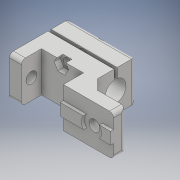
# Autodesk Inventor part: EixoXY - Canto
Saved by Autodesk Inventor 2017 (Build 210142000, 142)
## iProperties
Created: 2020-08-07
Part Number: EixoXY - Canto
Material: Generic
Document SubType Name: Modeling
Designer: ale
Density: 1 g/cm^3
Appearance: Default
Author: ale
Autodesk Inventor part; units mm, degrees
note: some values were not read from the file. Chosen so that the rebuilt part matches the saved one: direction of "Hole1".
ref_plane "YZ Plane" through (0, 0, 0) normal (1, 0, 0) x (0, 1, 0)
ref_plane "XZ Plane" through (0, 0, 0) normal (0, 1, 0) x (-1, 0, 0)
ref_plane "XY Plane" through (0, 0, 0) normal (0, 0, 1) x (1, 0, 0)
sketch "Sketch2" plane through (0, 0, 0) normal (0, 0, 1) x (1, 0, 0)
  line L0 (0, 0) -> (0, -10)
  line L1 (0, 0) -> (-27, 0)
  line L2 (-27, 0) -> (-27, 20)
  line L3 (-27, 20) -> (6, 20)
  line L4 (0, -10) -> (25, -10)
  line L5 (25, -10) -> (25, -4)
  line L6 (25, -4) -> (6, -4)
  line L7 (6, 20) -> (6, -4)
  dimension "d4" = 10
  dimension "d5" = 27
  dimension "d6" = 20
  dimension "d7" = 33
  dimension "d9" = 25
  dimension "d10" = 6
  constraints: 16 end point, 5 perpendicular, 2 horizontal, 1 vertical
  measures "d4" distance of L0.start L0.end
  measures "d5" distance of L0.start L1.end
  measures "d6" distance of L1.end L2.end
  measures "d7" distance of L2.end L3.end
  measures "d9" distance of L0.end L4.end
  measures "d10" distance of L4.end L5.end
extrude "Extrusion6" add sketch "Sketch2" against normal blind 20
sketch "Sketch9" plane through (6, -4, 0) normal (1, 0, 0) x (0, 0, -1)
  line L0 (0, 4) -> (20, 4) projected
  line L1 (20, 24) -> (20, 0) projected
  line L2 (0, 4) -> (20, 24)
  arc A0 (4.8038, 13.25) -> (4.8038, 14.75) centre (10, 14) ccw
  line L3 (4.8038, 14.75) -> (0, 14.75)
  line L4 (4.8038, 13.25) -> (0, 13.25)
  line L5 (0, 13.25) -> (0, 14.75)
  line L6 (0, 0) -> (0, 24) projected
  dimension "d28" = 10.5
  constraints: 8 end point, 2 point on circle, 1 centre point, 1 collinear, 1 midpoint
  measures "d28" diameter of A0
extrude "Extrusion7" cut sketch "Sketch9" against normal through all contours A0 L4 L5 L3 L2 | L2 A0
sketch "Sketch10" plane through (-27, 0, 0) normal (0, -1, 0) x (1, 0, 0)
  line L0 (33, 0) -> (0, 0) projected
  line L1 (0, 0) -> (6, 0)
  line L2 (6, 0) -> (6, -20)
  line L3 (6, -20) -> (0, -20)
  line L4 (0, -20) -> (0, 0)
  point P0 (27, 0)
  dimension "d33" = 6
  dimension "d34" = 20
  constraints: 8 end point, 2 parallel, 1 horizontal, 1 perpendicular
  measures "d33" distance of L2.end L3.end
  measures "d34" distance of L1.end L2.end
extrude "Extrusion8" add sketch "Sketch10" along normal blind 10
sketch "Sketch11" plane through (-27, 20, -20) normal (-1, 0, 0) x (0, 0, 1)
  line L0 (20, -30) -> (0, -30) projected
  line L1 (20, -20) -> (20, -30) projected
  line L2 (0, -30) -> (20, -20)
  point P0 (10, -25)
  constraints: 2 end point, 1 midpoint
hole "Hole1" at (-27, -5, -10) direction (1, 0, 0) diameter 5.5 end up to surface
sketch "Sketch13" plane through (0, -10, 0) normal (0, -1, 0) x (1, 0, 0)
  line L0 (0, -13) -> (25, -13)
  line L1 (0, -7) -> (25, -7)
  line L2 (0, -13) -> (0, -7)
  line L3 (0, 0) -> (0, -20) projected
  line L4 (25, -7) -> (25, -13)
  line L5 (0, 0) -> (25, 0) projected
  dimension "d69" = 25
  constraints: 8 end point, 1 collinear, 1 perpendicular
  measures "d69" distance between parallel lines of L4 L3
extrude "Extrusion9" add sketch "Sketch13" along normal blind 1.5
sketch "Sketch14" plane through (0, -11.5, 0) normal (0, -1, 0) x (1, 0, 0)
  line L0 (0, -7) -> (25, -7) projected
  line L1 (25, -13) -> (0, -13) projected
  line L2 (0, -13) -> (25, -13) projected
  line L3 (25, 0) -> (25, -7) projected
  point P0 (0, 0)
  point P1 (15.5, -10)
  dimension "d70" = 9.5
  measures "d70" distance from line of L3 point (15.5, -10)
hole "Hole2" at (15.5, -11.5, -10) direction (0, 1, 0) diameter 5.5 end through all counterbore diameter 10 counterbore depth 1.5
sketch "Sketch15" plane through (-27, 20, 0) normal (0, 1, 0) x (1, 0, 0)
  line L0 (33, 4.8038) -> (0, 4.8038) projected
  point P0 (27, 0)
  point P1 (16, 2.4019)
hole "Hole3" at (-11, 20, -2.4019) direction (0, -1, 0) diameter 4 end through all
sketch "Sketch16" plane through (0, 0, -20) normal (0, -1, 0) x (1, 0, 0)
  circle A0 centre (-11, 17.5981) radius 2 projected
  line L0 (-7.4, 17.6276) -> (-9.1744, 14.4952)
  line L1 (-9.1744, 14.4952) -> (-12.7744, 14.4656)
  line L2 (-12.7744, 14.4656) -> (-14.6, 17.5685)
  line L3 (-14.6, 17.5685) -> (-12.8256, 20.701)
  line L4 (-12.8256, 20.701) -> (-9.2256, 20.7305)
  line L5 (-9.2256, 20.7305) -> (-7.4, 17.6276)
  point P0 (0, 20)
  point P1 (-11, 17.5981)
  dimension "d65" = 7.2
  constraints: 12 end point, 1 coincident, 13 other
  measures "d65" horizontal distance of L2.end L0.start
extrude "Extrusion10" cut sketch "Sketch16" against normal blind 3
fillet "Fillet2" radius 2 9 edges at (-24, -10, 0) (-24, -10, -20) (-27, 20, -10) (6, 20, -10) (-10.5, 20, -20) (-10.5, 20, 0) (25, -7, -20) (25, -4, -10) (25, -7, 0)
chamfer "Chamfer3" distance 5 angle 45 1 edges at (6, -4, -10)
body "Solid3"
